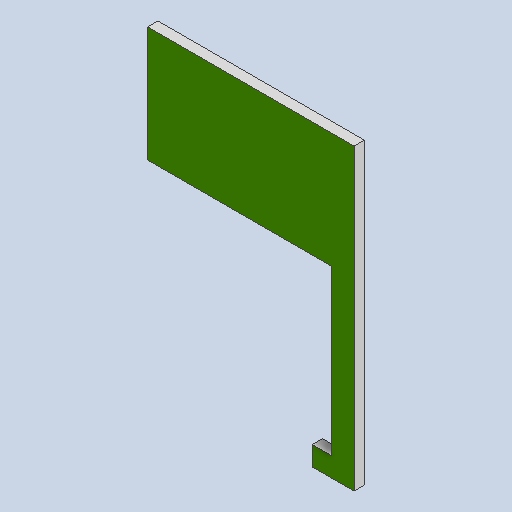
# Autodesk Inventor part: PCB_2_Miras
Saved by Autodesk Inventor 2023 (Build 270158000, 158)
## iProperties
Created: 2023-01-03
Part Number: PCB_2_Miras
Material: Generic
Document SubType Name: Modeling
Designer: Kamil
Density: 1 g/cm^3
Appearance: Default
Author: Kamil
Autodesk Inventor part; units mm, degrees
ref_plane "YZ Plane" through (0, 0, 0) normal (1, 0, 0) x (0, 1, 0)
ref_plane "XZ Plane" through (0, 0, 0) normal (0, 1, 0) x (-1, 0, 0)
ref_plane "XY Plane" through (0, 0, 0) normal (0, 0, 1) x (1, 0, 0)
sketch "Sketch1" plane through (0, 0, 0) normal (0, 0, 1) x (1, 0, 0)
  line L0 (12.5, -5.24) -> (15, -5.24) projected
  line L1 (15, -5.24) -> (15, -10.24) projected
  line L2 (15, -10.24) -> (12.5, -10.24) projected
  arc A0 (12.5, -5.24) -> (12.5, -10.24) centre (12.5, -7.74) ccw projected
  line L3 (-15, -5.24) -> (-12.5, -5.24) projected
  arc A1 (-12.5, -10.24) -> (-12.5, -5.24) centre (-12.5, -7.74) ccw projected
  line L4 (-12.5, -10.24) -> (-15, -10.24) projected
  line L5 (-15, -10.24) -> (-15, -5.24) projected
  circle A2 centre (-7.5, -12.2) radius 1.75 projected
  circle A3 centre (7.5, -12.2) radius 1.75 projected
  line L6 (2.4, 25.954) -> (2.4, 24.254) projected
  line L7 (4, 25.954) -> (2.4, 25.954) projected
  line L8 (4, 24.254) -> (4, 25.954) projected
  line L9 (50, 22.6643) -> (44, 22.6643) projected
  line L10 (44, 22.6643) -> (44, -4.7413) projected
  arc A4 (44, -9.7413) -> (44, -4.7413) centre (44, -7.2413) ccw projected
  line L11 (44, -9.7413) -> (44, -18.8012) projected
  line L12 (44, -18.8012) -> (50, -18.8012) projected
  line L13 (50, -18.8012) -> (50, 22.6643) projected
  line L14 (40.2471, -8.6254) -> (44, -18.8012) projected
  line L15 (44, -9.7413) -> (44, -18.8012) projected
  arc A5 (44, -4.7413) -> (44, -9.7413) centre (44, -7.2413) ccw projected
  line L16 (44, 4.3187) -> (44, -4.7413) projected
  line L17 (44, 4.3187) -> (40.2471, -5.8572) projected
  arc A6 (40.2471, -5.8572) -> (40.2471, -8.6254) centre (44, -7.2413) ccw projected
  line L18 (8.95, 13.1005) -> (37.5, 13.1005)
  line L19 (37.5, 13.1005) -> (37.5, 31.0066)
  line L20 (37.5, 31.0066) -> (8.95, 31.0066)
  line L21 (8.95, 31.0066) -> (8.95, 13.1005)
  line L22 (44, 18.1772) -> (41, 18.1772)
  line L23 (41, 18.1772) -> (41, 7.8033)
  line L24 (41, 7.8033) -> (44, 7.8033)
  line L25 (44, 7.8033) -> (44, 18.1772)
  line L26 (37.5, 31.0066) -> (41, 31.0066)
  line L27 (41, 31.0066) -> (41, 1.9316)
  line L28 (41, 1.9316) -> (37.5, 1.9316)
  line L29 (37.5, 1.9316) -> (37.5, 31.0066)
  line L30 (8.95, 31.0066) -> (41, 31.0066)
  line L31 (41, 31.0066) -> (41, 23.254)
  line L32 (41, 23.254) -> (8.95, 23.254)
  line L33 (8.95, 23.254) -> (8.95, 31.0066)
  line L34 (17.8602, 13.1005) -> (37.5, 13.1005)
  line L35 (37.5, 13.1005) -> (37.5, -15.4)
  line L36 (37.5, -15.4) -> (17.8602, -15.4)
  line L37 (17.8602, -15.4) -> (17.8602, 13.1005)
  line L38 (37.5, -15.4) -> (41, -15.4)
  line L39 (41, -15.4) -> (41, 1.9316)
  line L40 (41, 1.9316) -> (37.5, 1.9316)
  line L41 (37.5, 1.9316) -> (37.5, -15.4)
  arc A7 (-17.7252, -6.9095) -> (-17.704, -4.5096) centre (-17.7146, -5.7096) ccw projected
  line L42 (-17.7252, -6.9095) -> (-18.8252, -6.8998) projected
  arc A8 (-18.8039, -4.4999) -> (-18.8252, -6.8998) centre (-18.8145, -5.6998) ccw projected
  line L43 (-18.8039, -4.4999) -> (-17.704, -4.5096) projected
  circle A9 centre (21.3634, 8.1005) radius 1.5 projected
  arc A10 (-17.5172, 16.5895) -> (-17.496, 18.9894) centre (-17.5066, 17.7895) ccw projected
  line L44 (-17.5172, 16.5895) -> (-18.6172, 16.5993) projected
  arc A11 (-18.5959, 18.9992) -> (-18.6172, 16.5993) centre (-18.6065, 17.7992) ccw projected
  line L45 (-18.5959, 18.9992) -> (-17.496, 18.9894) projected
  circle A12 centre (34, -10.4) radius 1.5 projected
  arc A13 (36.5, 15.1772) -> (34.5, 17.1772) centre (34.5, 15.1772) ccw projected
  line L46 (16.4051, 17.1772) -> (34.5, 17.1772) projected
  arc A14 (12.4051, 21.1772) -> (16.4051, 17.1772) centre (16.4051, 21.1772) ccw projected
  line L47 (12.4051, 28.0066) -> (12.4051, 21.1772) projected
  arc A15 (12.4051, 28.0066) -> (10.4051, 30.0066) centre (10.4051, 28.0066) ccw projected
  line L48 (-18.5665, 30.0066) -> (10.4051, 30.0066) projected
  arc A16 (-18.5665, 30.0066) -> (-20.5665, 28.0066) centre (-18.5665, 28.0066) ccw projected
  line L49 (-20.5665, 18.4539) -> (-20.5665, 28.0066) projected
  arc A17 (-24.5665, 14.4539) -> (-20.5665, 18.4539) centre (-24.5665, 18.4539) ccw projected
  line L50 (-34.5, 14.4539) -> (-24.5665, 14.4539) projected
  arc A18 (-34.5, 14.4539) -> (-36.5, 12.4539) centre (-34.5, 12.4539) ccw projected
  line L51 (-36.5, -12.4) -> (-36.5, 12.4539) projected
  arc A19 (-36.5, -12.4) -> (-34.5, -14.4) centre (-34.5, -12.4) ccw projected
  line L52 (34.5, -14.4) -> (-34.5, -14.4) projected
  arc A20 (34.5, -14.4) -> (36.5, -12.4) centre (34.5, -12.4) ccw projected
  line L53 (36.5, 15.1772) -> (36.5, -12.4) projected
  line L54 (5.95, 24.254) -> (4, 24.254) projected
  arc A21 (9.95, 20.254) -> (5.95, 24.254) centre (5.95, 20.254) ccw projected
  line L55 (9.95, 16.1005) -> (9.95, 20.254) projected
  arc A22 (9.95, 16.1005) -> (11.95, 14.1005) centre (11.95, 16.1005) ccw projected
  line L56 (14.8602, 14.1005) -> (11.95, 14.1005) projected
  arc A23 (18.8602, 10.1005) -> (14.8602, 14.1005) centre (14.8602, 10.1005) ccw projected
  line L57 (18.8602, -0.2) -> (18.8602, 10.1005) projected
  arc A24 (14.8602, -4.2) -> (18.8602, -0.2) centre (14.8602, -0.2) ccw projected
  line L58 (12.1354, -4.2) -> (14.8602, -4.2) projected
  arc A25 (12.1354, -4.2) -> (11.1485, -4.4605) centre (12.1354, -6.2) ccw projected
  line L59 (7.9105, -6.2976) -> (11.1485, -4.4605) projected
  arc A26 (5.9366, -6.8186) -> (7.9105, -6.2976) centre (5.9366, -2.8186) ccw projected
  line L60 (-5.9366, -6.8186) -> (5.9366, -6.8186) projected
  arc A27 (-7.9105, -6.2976) -> (-5.9366, -6.8186) centre (-5.9366, -2.8186) ccw projected
  line L61 (-11.1485, -4.4605) -> (-7.9105, -6.2976) projected
  arc A28 (-11.1485, -4.4605) -> (-12.1354, -4.2) centre (-12.1354, -6.2) ccw projected
  line L62 (-14.8602, -4.2) -> (-12.1354, -4.2) projected
  arc A29 (-18.8602, -0.2) -> (-14.8602, -4.2) centre (-14.8602, -0.2) ccw projected
  line L63 (-18.8602, 10.3433) -> (-18.8602, -0.2) projected
  arc A30 (-15.9867, 14.1814) -> (-18.8602, 10.3433) centre (-14.8602, 10.3433) ccw projected
  arc A31 (-15.9867, 14.1814) -> (-14.55, 16.1005) centre (-16.55, 16.1005) ccw projected
  line L64 (-14.55, 20.254) -> (-14.55, 16.1005) projected
  arc A32 (-10.55, 24.254) -> (-14.55, 20.254) centre (-10.55, 20.254) ccw projected
  line L65 (2.4, 24.254) -> (-10.55, 24.254) projected
  point P0 (0, 0)
  point P1 (41, -3.8157)
  point P2 (41, -10.6668)
  dimension "d0" = 3
  constraints: 48 end point, 12 parallel, 6 horizontal, 6 perpendicular, 2 point on line
  measures "d0" distance of L24.end L23.end
extrude "Extrusion1" add sketch "Sketch1" along normal blind 3.1 contours A21 L55 A22 L56 A23 L18 L21 | L21 L32 L47 A14 L46 A13 L53 L18 A23 L56 A22 L55 A21 | L21 L48 A15 L47 L32 | L21 L20 L19 L32 L47 A15 L48 | L32 L19 L18 L53 A13 L46 A14 L47 | L32 L27 L23 L28 L29 L19 | L19 L26 L27 L32
sketch "Sketch2" plane through (0, 0, 0) normal (0, 0, -1) x (-1, 0, 0)
  line L0 (-8.95, 31.0066) -> (-8.95, 13.1005) projected
  line L1 (-41, 1.9316) -> (-41, 31.0066) projected
  line L2 (-37.5, 1.9316) -> (-41, 1.9316) projected
  line L3 (-41, 31.0066) -> (-8.95, 31.0066) projected
  line L4 (-37.5, 13.1005) -> (-37.5, 1.9316) projected
  line L5 (-8.95, 13.1005) -> (-37.5, 13.1005) projected
  point P0 (0, 0)
extrude "Extrusion2" cut sketch "Sketch2" against normal blind 1.5
sketch "Sketch3" plane through (41, -3.8157, 3.1) normal (1, 0, 0) x (0, 0, -1)
  line L0 (38.317, 76.7923) -> (28.0867, 64.6003) projected
  line L1 (-3.9, -14.9855) -> (-3.9, 26.48) projected
  line L2 (-3.9, -14.9855) -> (7.1, -14.9855) projected
  line L3 (7.1, -14.9855) -> (7.1, 1.1145) projected
  arc A0 (25.2, 19.2145) -> (7.1, 1.1145) centre (25.2, 1.1145) ccw projected
  line L4 (25.2, 19.2145) -> (36.2, 19.2145) projected
  line L5 (1.6, 5.7473) -> (1.6, 34.8223) projected
  line L6 (1.6, 34.8223) -> (0, 34.8223) projected
  line L7 (0, 5.7473) -> (0, 34.8223) projected
  line L8 (0, 0) -> (0, 34.8223) projected
  line L9 (0, 30.197) -> (1.6, 30.197)
  line L10 (28.0867, 30.906) -> (23.6867, 30.906) projected
  line L11 (23.6867, 30.906) -> (23.6867, 44.6714) projected
  line L12 (23.6867, 44.6714) -> (28.0867, 44.6714) projected
  line L13 (28.0867, 44.6714) -> (28.0867, 30.906) projected
  line L14 (28.0867, 64.6003) -> (28.0867, 59.2448) projected
  line L15 (36.2, 19.2145) -> (36.2, 63.075) projected
  line L16 (36.2, 63.075) -> (39.2, 63.075) projected
  line L17 (39.2, 63.075) -> (39.2, 76.4709) projected
  line L18 (23.5929, 59.2448) -> (-3.9, 26.48) projected
  arc A1 (39.2, 76.4709) -> (38.317, 76.7923) centre (38.7, 76.4709) ccw projected
  line L19 (23.5929, 59.2448) -> (28.0867, 59.2448) projected
  line L20 (11.8485, 39.6478) -> (14.4531, 37.4623) projected
  line L21 (14.4531, 37.4623) -> (10.9819, 33.3255) projected
  line L22 (10.9819, 33.3255) -> (8.3773, 35.511) projected
  line L23 (11.8485, 39.6478) -> (8.3773, 35.511) projected
  line L24 (1.6, 5.7473) -> (0, 5.7473) projected
  point P0 (3.1, 3.8157)
  point P1 (36.2, 74.2694)
  constraints: 2 end point, 2 point on line, 1 perpendicular
extrude "Extrusion3" [suppressed]
sketch "Sketch4" plane through (0, 0, 3.1) normal (0, 0, 1) x (1, 0, 0)
  line L0 (31.7, -15.7) -> (31.7, 9.3) projected
  line L1 (41, -15.4) -> (41, -10.6668) projected
  line L2 (41, -3.8157) -> (41, -10.6668)
  line L3 (37.5, 1.9316) -> (41, 1.9316) projected
  line L4 (41, 31.0066) -> (8.95, 31.0066) projected
  line L5 (8.95, 31.0066) -> (8.95, 13.1005) projected
  line L6 (8.95, 13.1005) -> (37.5, 13.1005) projected
  line L7 (37.5, 13.1005) -> (37.5, 1.9316) projected
  line L8 (41, 1.9316) -> (41, 31.0066) projected
  point P0 (0, 0)
  constraints: 2 end point
extrude "Extrusion4" [suppressed]
sketch "Sketch5" plane through (0, 0, 3.1) normal (0, 0, 1) x (1, 0, 0)
  line L0 (15, 8.3373) -> (15, -1.2152) projected
  line L1 (8.95, 13.1005) -> (17.8602, 13.1005) projected
  line L2 (17.8602, 13.1005) -> (16.3634, 13.1005)
  line L3 (16.3634, 13.1005) -> (16.3634, -15.4)
  line L4 (16.3634, -15.4) -> (17.8602, -15.4)
  line L5 (17.8602, -15.4) -> (17.8602, 13.1005)
  line L6 (37.5, 1.9316) -> (41, 1.9316) projected
  line L7 (41, 31.0066) -> (8.95, 31.0066) projected
  line L8 (8.95, 31.0066) -> (8.95, 13.1005) projected
  line L9 (8.95, 13.1005) -> (37.5, 13.1005) projected
  line L10 (37.5, 13.1005) -> (37.5, 1.9316) projected
  line L11 (41, 1.9316) -> (41, 31.0066) projected
  point P0 (0, 0)
  constraints: 8 end point, 2 parallel, 1 horizontal, 1 perpendicular
extrude "Extrusion5" [suppressed]
sketch "Sketch6" plane through (0, 0, 3.1) normal (0, 0, 1) x (1, 0, 0)
  line L0 (16.3634, -15.4) -> (41, -15.4) projected
  line L1 (28.6817, -15.4) -> (28.6817, 26.3813)
  line L2 (41, 26.3813) -> (8.95, 26.3813) projected
  line L3 (28.6817, -15.4) -> (28.6817, -9.9)
  line L4 (28.6817, 26.3813) -> (28.6817, 20.8813)
  line L5 (16.3634, 13.1005) -> (41, 13.1005)
  line L6 (41, -15.4) -> (41, 26.3813) projected
  line L7 (16.3634, 13.1005) -> (21.3634, 13.1005)
  line L8 (21.3634, 13.1005) -> (21.3634, 8.1005)
  line L9 (21.3634, 8.1005) -> (16.3634, 8.1005)
  line L10 (16.3634, 8.1005) -> (16.3634, 13.1005)
  line L11 (41, -15.4) -> (36, -15.4)
  line L12 (36, -15.4) -> (36, -10.4)
  line L13 (36, -10.4) -> (41, -10.4)
  line L14 (41, -10.4) -> (41, -15.4)
  circle A0 centre (21.3634, 8.1005) radius 1.5
  circle A1 centre (36, -10.4) radius 1.5
  line L15 (37.5, 1.9316) -> (41, 1.9316) projected
  line L16 (41, 31.0066) -> (8.95, 31.0066) projected
  line L17 (8.95, 31.0066) -> (8.95, 13.1005) projected
  line L18 (8.95, 13.1005) -> (37.5, 13.1005) projected
  line L19 (37.5, 13.1005) -> (37.5, 1.9316) projected
  line L20 (41, 1.9316) -> (41, 31.0066) projected
  point P0 (0, 0)
  dimension "d11" = 5.5
  dimension "d12" = 5.5
  dimension "d13" = 5
  dimension "d14" = 5
  dimension "d15" = 5
  dimension "d16" = 5
  dimension "d17" = 3
  dimension "d18" = 3
  constraints: 24 end point, 4 parallel, 4 point on line, 2 centre point, 2 coincident, 2 horizontal, 2 perpendicular, 1 midpoint
  measures "d11" distance of L1.start L3.end
  measures "d12" distance of L1.end L4.end
  measures "d13" distance of L8.end L9.end
  measures "d14" distance of L7.end L8.end
  measures "d15" distance of L12.end L13.end
  measures "d16" distance of L11.end L12.end
  measures "d17" diameter of A0
  measures "d18" diameter of A1
extrude "Extrusion6" cut sketch "Sketch6" against normal blind 1.6 contours A1 L13 L12 | L12 L13 A1 | A0 L9 L8 | L8 L9 A0
sketch "Sketch8" plane through (0, 0, 3.1) normal (0, 0, 1) x (1, 0, 0)
  line L0 (36, -10.4) -> (34, -10.4)
  circle A0 centre (34, -10.4) radius 1.5
  line L1 (37.5, 1.9316) -> (41, 1.9316) projected
  line L2 (41, 31.0066) -> (8.95, 31.0066) projected
  line L3 (8.95, 31.0066) -> (8.95, 13.1005) projected
  line L4 (8.95, 13.1005) -> (37.5, 13.1005) projected
  line L5 (37.5, 13.1005) -> (37.5, 1.9316) projected
  line L6 (41, 1.9316) -> (41, 31.0066) projected
  point P0 (0, 0)
  dimension "d21" = 2
  constraints: 2 end point, 1 centre point, 1 coincident, 1 horizontal
  measures "d21" distance of L0.start L0.end
extrude "Extrusion7" [suppressed]
extrude "Extrusion8" cut sketch "Sketch8" against normal blind 1.6 contours A0
sketch "Sketch9" plane through (0, 0, 3.1) normal (0, 0, 1) x (1, 0, 0)
  line L0 (37.5, 1.9316) -> (41, 1.9316) projected
  line L1 (8.95, 13.1005) -> (41, 13.1005)
  line L2 (41, 13.1005) -> (41, 26.3813)
  line L3 (41, 26.3813) -> (8.95, 26.3813)
  line L4 (8.95, 26.3813) -> (8.95, 13.1005)
  line L5 (41, 31.0066) -> (8.95, 31.0066) projected
  line L6 (8.95, 31.0066) -> (8.95, 13.1005) projected
  line L7 (8.95, 13.1005) -> (37.5, 13.1005) projected
  line L8 (37.5, 13.1005) -> (37.5, 1.9316) projected
  line L9 (41, 1.9316) -> (41, 31.0066) projected
  point P0 (0, 0)
  constraints: 8 end point, 2 parallel, 1 horizontal, 1 perpendicular
extrude "Extrusion9" [suppressed]
sketch "Sketch10" plane through (0, 0, 3.1) normal (0, 0, 1) x (1, 0, 0)
  line L0 (37.5, 1.9316) -> (41, 1.9316) projected
  line L1 (41, 1.9316) -> (37.5, 1.9316)
  line L2 (37.5, 1.9316) -> (37.5, -15.4)
  line L3 (37.5, -15.4) -> (41, -15.4)
  line L4 (41, -15.4) -> (41, 1.9316)
  arc A0 (34.5, -15.4) -> (37.5, -12.4) centre (34.5, -12.4) ccw projected
  line L5 (37.5, -15.4) -> (34.5, -15.4)
  line L6 (34.5, -15.4) -> (34.5, -12.4)
  line L7 (34.5, -12.4) -> (37.5, -12.4)
  line L8 (37.5, -12.4) -> (37.5, -15.4)
  line L9 (41, 31.0066) -> (8.95, 31.0066) projected
  line L10 (8.95, 31.0066) -> (8.95, 13.1005) projected
  line L11 (8.95, 13.1005) -> (37.5, 13.1005) projected
  line L12 (37.5, 13.1005) -> (37.5, 1.9316) projected
  line L13 (41, 1.9316) -> (41, 31.0066) projected
  point P0 (0, 0)
  constraints: 16 end point, 4 parallel, 2 horizontal, 2 perpendicular
extrude "Extrusion10" add sketch "Sketch10" against normal blind 1.6 contours L0 L4 L3 L2 | L2 L5 A0 | A0 L6 L7
body "Solid1"
